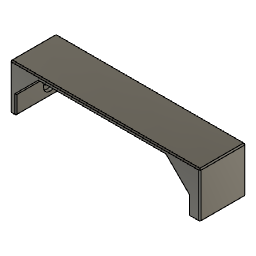
Electronics Base v1 (Autodesk Fusion 360 design; units mm, degrees)
Autodesk Fusion 360 part; units mm, degrees
note: some values were not read from the file. Set by a fixed rule: which sketch regions a step uses.
sketch "Sketch1" plane through (0, 0, 0) normal (1, 0, 0) x (0, 1, 0)
  line L0 (20, 20) -> (-20, 20)
  line L1 (-20, 20) -> (-20, -20)
  line L2 (-20, -20) -> (20, -20)
  line L3 (20, -20) -> (20, 20)
  line L4 (20, 20) -> (-20, -20) construction
  line L5 (-20, 20) -> (20, -20) construction
  line L6 (10, 10) -> (-10, 10) construction
  line L7 (-10, 10) -> (-10, -10) construction
  line L8 (-10, -10) -> (10, -10) construction
  line L9 (10, -10) -> (10, 10) construction
  line L10 (10, 10) -> (-10, -10) construction
  line L11 (-10, 10) -> (10, -10) construction
  circle A0 centre (-10, 10) radius 2.75
  circle A1 centre (10, -10) radius 2.75
  dimension "d3" = 40
  dimension "d5" = 5.5
  dimension "d6" = 20
  dimension "d12" = 40
  constraint horizontal L0
  constraint perpendicular L0 L1
  constraint parallel L0 L2
  constraint parallel L1 L3
  constraint coincident L4 origin
  constraint coincident L5 origin
  constraint horizontal L6
  constraint perpendicular L6 L7
  constraint parallel L6 L8
  constraint parallel L7 L9
  constraint coincident L4 L6.start
  constraint coincident L10 origin
  constraint coincident L11 origin
  constraint coincident L6.end L7.start
  constraint coincident L8.end L9.start
  measures "d3" distance of L0.start L0.end
  measures "d5" diameter of A0
  measures "d6" distance of L6.start L6.end
  measures "d12" distance of L0.end L1.end
extrude "Extrude1" add sketch "Sketch1" along normal blind 5
sketch "Sketch2" plane through (5, 0, 0) normal (1, 0, 0) x (0, 1, 0)
  circle A0 centre (10, -10) radius 2.75
  circle A1 centre (-10, 10) radius 2.75
  line L0 (20, -20) -> (20, 20)
  line L1 (20, 20) -> (-20, 20)
  line L2 (-20, 20) -> (-20, -20)
  line L3 (-20, -20) -> (20, -20)
  circle A2 centre (-10, 10) radius 6
  circle A3 centre (10, -10) radius 6
  dimension "d9" = 12
  constraint concentric A1 A2
  constraint concentric A0 A3
  measures "d9" diameter of A2
extrude "Extrude2" cut sketch "Sketch2" against normal blind 3 contours A2 | A3
sketch "Sketch3" plane through (5, 0, 0) normal (1, 0, 0) x (0, 1, 0)
  circle A0 centre (-10, 10) radius 6
  circle A1 centre (10, -10) radius 6
  line L0 (20, -20) -> (20, 20)
  line L1 (20, 20) -> (-20, 20)
  line L2 (-20, 20) -> (-20, -20)
  line L3 (-20, -20) -> (20, -20)
  line L4 (-20, 20) -> (20, 20)
  line L5 (20, 20) -> (20, 16)
  line L6 (20, 16) -> (-20, 16)
  line L7 (-20, 16) -> (-20, 20)
  dimension "d13" = 4
  constraint horizontal L4
  constraint vertical L5
  constraint horizontal L6
  constraint vertical L7
  constraint coincident L0 L5.end
  constraint coincident L1.end L2.start
  measures "d13" distance of L0.end L5.end
extrude "Extrude3" add sketch "Sketch3" along normal blind 160.2 contours L0 L1 L2 L4 L5 L6 L7
sketch "Sketch4" plane through (0, 0, 16) normal (0, 0, -1) x (1, 0, 0)
  line L0 (5, 10) -> (5, -20)
  line L1 (5, -20) -> (165.2, -20)
  line L2 (165.2, -20) -> (165.2, 20)
  line L3 (165.2, 20) -> (5, 20)
  line L4 (165.2, 20) -> (155.2, 20)
  line L5 (155.2, 20) -> (155.2, -20)
  line L6 (155.2, -20) -> (165.2, -20)
  line L7 (165.2, -20) -> (165.2, 20)
  line L8 (5, 20) -> (5, 10)
  dimension "d16" = 10
  constraint horizontal L4
  constraint vertical L5
  constraint horizontal L6
  constraint vertical L7
  constraint coincident L1 L5.end
  constraint coincident L2.end L3.start
  measures "d16" distance of L5.end L1.end
extrude "Extrude4" add sketch "Sketch4" along normal up to surface (36 mm away) contours L1 L2 L3 L4 L5 L6 L7
sketch "Sketch5" plane through (0, 20, 0) normal (0, 1, 0) x (-1, 0, 0)
  line L0 (0, -20) -> (0, 20)
  line L1 (0, 20) -> (-165.2, 20)
  line L2 (-165.2, 20) -> (-165.2, -20)
  line L3 (-165.2, -20) -> (-155.2, -20)
  line L4 (-155.2, -20) -> (-155.2, 16)
  line L5 (-155.2, 16) -> (-5, 16)
  line L6 (-5, 16) -> (-5, -20)
  line L7 (-5, -20) -> (0, -20)
  line L8 (-25, 16) -> (-5, -4)
  line L9 (-5, 16) -> (-25, 16)
  line L10 (-5, 16) -> (-5, -4)
  line L11 (-155.2, 16) -> (-135.2, 16)
  line L12 (-155.2, 16) -> (-155.2, -4)
  line L13 (-155.2, -4) -> (-135.2, 16)
  dimension "d19" = 20
  dimension "d22" = 20
  constraint coincident L5 L8.start
  constraint coincident L6 L8.end
  constraint coincident L5.end L6.start
  constraint perpendicular L6 L9
  constraint equal L9 L10
  constraint coincident L8.start L9.end
  constraint coincident L4.end L5.start
  constraint coincident L5 L11.end
  constraint coincident L4 L12.end
  constraint perpendicular L11 L12
  constraint equal L11 L12
  measures "d19" distance of L8.start L5.end
  measures "d22" distance of L4.end L11.end
extrude "Extrude5" add sketch "Sketch5" against normal blind 5 contours L5 L6 L8 L9 L10 | L4 L5 L11 L12 L13
mirror "Mirror1" about plane through (0, 0, 0) normal (0, 1, 0) of "Extrude5"
chamfer "Chamfer1" distance 1 angle 45 7 edges at (155.2, 0, -20) (145.2, -15, 6) (145.2, 15, 6) (15, -15, 6) (15, 15, 6) (5, 0, -20) (0, 0, 20) 3 faces at (165.2, 6.6667, -6.6667) (151.8667, -20, 10.6667) (151.8667, 20, 10.6667)
